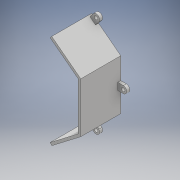
# Autodesk Inventor part: Capcture Zone4
Saved by Autodesk Inventor 2018 (Build 220112000, 112)
## iProperties
Created: 2017-10-26
Part Number: Capcture Zone4
Material: Generic
Document SubType Name: Modeling
Designer: Matthew Feros
Density: 1 g/cm^3
Appearance: Default
Author: Matthew Feros
Autodesk Inventor part; units mm, degrees
ref_plane "YZ Plane" through (0, 0, 0) normal (1, 0, 0) x (0, 1, 0)
ref_plane "XZ Plane" through (0, 0, 0) normal (0, 1, 0) x (-1, 0, 0)
ref_plane "XY Plane" through (0, 0, 0) normal (0, 0, 1) x (1, 0, 0)
sketch "Sketch1" plane through (0, 0, 0) normal (0, 1, 0) x (-1, 0, 0)
  line L0 (0, 0) -> (0, 23.8143)
  line L1 (0, 23.8143) -> (7.4151, 29.5041)
  line L2 (0, 23.8143) -> (9.3465, 23.8143) construction
  line L3 (0, 23.8143) -> (28, 45.2994)
  line L4 (0, 23.8143) -> (0, -23.8137)
  line L5 (0, -23.8137) -> (28, -45.2989)
  line L6 (28, -45.2989) -> (26.4781, -47.2823)
  line L7 (26.4781, -47.2823) -> (-0.4066, -26.6529)
  line L8 (0, -16.592) -> (-2.5, -16.592)
  line L9 (-2.5, -16.592) -> (-2.5, -25.0466)
  line L10 (-2.5, -25.0466) -> (-0.4066, -26.6529)
  line L11 (-2.5, -16.592) -> (-2.5, 22.9887)
  line L12 (0.8654, 24.4783) -> (-0.6565, 26.4617)
  line L13 (-0.6565, 26.4617) -> (-2.5, 25.0471)
  line L14 (-2.5, 25.0471) -> (-2.5, 22.9887)
  line L15 (-0.6565, 26.4617) -> (26.4781, 47.2828)
  line L16 (26.4781, 47.2828) -> (28, 45.2994)
  line L17 (26.4781, 47.2828) -> (28, 45.2994)
  line L18 (28, 45.2994) -> (0.8654, 24.4783)
  dimension "d0" = 23.8143
  dimension "d1" = 37.5
  dimension "d2" = 35.2932
  dimension "d3" = 47.628
  dimension "d4" = 35.2932
  dimension "d5" = 2.5
  dimension "d6" = 2.5
  dimension "d7" = 2.5
  constraints: 38 end point, 7 perpendicular, 6 point on line, 2 collinear, 2 vertical, 1 equal length, 1 horizontal
  measures "d0" distance of L0.start L0.end
  measures "d1" angle of L2 L1
  measures "d2" distance of L0.end L3.end
  measures "d3" distance of L0.end L4.end
  measures "d4" distance of L4.end L5.end
  measures "d5" distance of L5.end L6.end
  measures "d6" distance of L8.start L8.end
  measures "d7" distance of L12.start L12.end
extrude "Extrusion1" add sketch "Sketch1" along normal blind 40
sketch "Sketch2" plane through (0, 40, 0) normal (0, 1, 0) x (1, 0, 0)
  line L0 (0, 0) -> (8, 0)
  line L1 (-28, 45.2989) -> (0, 23.8137) projected
  line L2 (-28, 45.2989) -> (-24.0332, 42.2551)
  line L3 (-24.0332, 42.2551) -> (-19.1631, 48.6019)
  line L4 (0, -23.8143) -> (-28, -45.2994) projected
  line L5 (-28, -45.2994) -> (-24.0332, -42.2556)
  line L6 (-24.0332, -42.2556) -> (-19.1631, -48.6024)
  circle A0 centre (-19.1631, -48.6024) radius 1.75
  circle A1 centre (-19.1631, -48.6024) radius 3.5
  circle A2 centre (8, 0) radius 1.75
  circle A3 centre (8, 0) radius 3.5
  circle A4 centre (-19.1631, 48.6019) radius 1.75
  circle A5 centre (-19.1631, 48.6019) radius 3.5
  line L7 (2.5, 25.0466) -> (-26.4781, 47.2823) projected
  line L8 (-22.5113, 44.2385) -> (-25.2881, 46.3691)
  line L9 (-25.2881, 46.3691) -> (-21.9399, 50.7326)
  line L10 (-22.5113, 44.2385) -> (-19.7346, 42.1078)
  line L11 (-19.7346, 42.1078) -> (-16.3864, 46.4712)
  line L12 (8, 3.5) -> (2.5, 3.5)
  line L13 (2.5, 3.5) -> (2.5, -3.5)
  line L14 (2.5, -25.0471) -> (2.5, 25.0466) projected
  line L15 (2.5, -3.5) -> (8, -3.5)
  line L16 (-26.4781, -47.2828) -> (2.5, -25.0471) projected
  line L17 (-22.5113, -44.239) -> (-19.7346, -42.1083)
  line L18 (-19.7346, -42.1083) -> (-16.3864, -46.4718)
  line L19 (-22.5113, -44.239) -> (-25.2881, -46.3697)
  line L20 (-25.2881, -46.3697) -> (-21.9399, -50.7331)
  dimension "d10" = 8
  dimension "d11" = 5
  dimension "d12" = 8
  dimension "d13" = 8
  dimension "d14" = 3.5
  dimension "d15" = 7
  dimension "d16" = 3.5
  dimension "d17" = 7
  dimension "d18" = 3.5
  dimension "d19" = 7
  dimension "d20" = 3.5
  dimension "d21" = 3.5
  constraints: 32 end point, 11 point on line, 7 perpendicular, 6 centre point, 6 coincident, 6 point on circle, 2 horizontal
  measures "d10" distance of L0.start L0.end
  measures "d11" distance of L1.start L2.end
  measures "d12" distance of L2.end L3.end
  measures "d13" distance of L5.end L6.end
  measures "d14" diameter of A0
  measures "d15" diameter of A1
  measures "d16" diameter of A2
  measures "d17" diameter of A3
  measures "d18" diameter of A4
  measures "d19" diameter of A5
  measures "d20" distance of L8.start L8.end
  measures "d21" distance of L8.start L10.end
extrude "Extrusion2" add sketch "Sketch2" against normal blind 3
sketch "Sketch3" plane through (0, 0, 0) normal (0, -1, 0) x (1, 0, 0)
  line L0 (0, 0) -> (0, 10)
  line L1 (0, -23.8137) -> (0, 23.8143) projected
  line L2 (0, 10) -> (0, -10)
  line L3 (0, -10) -> (8, -10)
  line L4 (0, 10) -> (8, 10)
  circle A0 centre (8, 10) radius 1.75
  circle A1 centre (8, -10) radius 1.75
  circle A2 centre (8, -10) radius 3.5
  circle A3 centre (8, 10) radius 3.5
  line L5 (2.5, 25.0471) -> (2.5, -25.0466) projected
  line L6 (2.5, 10) -> (2.5, 6.5)
  line L7 (2.5, 6.5) -> (8, 6.5)
  line L8 (2.5, 10) -> (2.5, 13.5)
  line L9 (2.5, 13.5) -> (8, 13.5)
  line L10 (2.5, -10) -> (2.5, -13.5)
  line L11 (2.5, -13.5) -> (8, -13.5)
  line L12 (2.5, -10) -> (2.5, -6.5)
  line L13 (2.5, -6.5) -> (8, -6.5)
  dimension "d24" = 10
  dimension "d25" = 20
  dimension "d26" = 8
  dimension "d27" = 3.5
  dimension "d28" = 7
  constraints: 24 end point, 10 point on line, 5 perpendicular, 4 centre point, 4 coincident, 4 point on circle, 1 horizontal
  measures "d24" distance of L0.start L0.end
  measures "d25" distance of L0.end L2.end
  measures "d26" distance of L2.end L3.end
  measures "d27" diameter of A0
  measures "d28" diameter of A2
extrude "Extrusion3" add sketch "Sketch3" against normal blind 3 contours L5 L9 A3 L4 | L4 A3 L7 L5 | L5 L13 A2 L3 | L3 A2 L11 L5 | A3 | A2
sketch "Sketch4" plane through (0, 0, 0) normal (0, -1, 0) x (1, 0, 0)
  line L0 (2.5, 13.5) -> (8, 13.5) projected
  line L1 (2.5, 13.5) -> (12.0473, 13.5)
  line L2 (12.0473, 13.5) -> (12.0473, 6.5)
  line L3 (12.0473, 6.5) -> (2.5, 6.5)
  line L4 (2.5, 6.5) -> (2.5, 13.5)
  line L5 (2.5, -6.5) -> (8, -6.5) projected
  line L6 (2.5, -6.5) -> (13.899, -6.5)
  line L7 (13.899, -6.5) -> (13.899, -13.5)
  line L8 (13.899, -13.5) -> (2.5, -13.5)
  line L9 (2.5, -13.5) -> (2.5, -6.5)
  point P0 (0, 0)
  dimension "d31" = 7
  constraints: 16 end point, 4 parallel, 2 horizontal, 2 perpendicular
  measures "d31" distance of L6.end L7.end
extrude "Extrusion4" cut sketch "Sketch4" against normal blind 3
body "Solid1"
